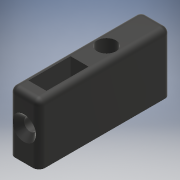
# Autodesk Inventor part: hotend__belt_holder
Saved by Autodesk Inventor 2018 (Build 220112000, 112)
## iProperties
Created: 2018-07-17
Part Number: hotend__belt_holder
Material: ABS Plastic
Document SubType Name: Modeling
Designer: Z. Deniz
Density: 1.06 g/cm^3
Appearance: Smooth - White
Author: Z. Deniz
Autodesk Inventor part; units mm, degrees
ref_plane "YZ Plane" through (0, 0, 0) normal (1, 0, 0) x (0, 1, 0)
ref_plane "XZ Plane" through (0, 0, 0) normal (0, 1, 0) x (-1, 0, 0)
ref_plane "XY Plane" through (0, 0, 0) normal (0, 0, 1) x (1, 0, 0)
sketch "Sketch1" plane through (0, 0, 0) normal (0, 0, 1) x (1, 0, 0)
  line L0 (0, 0) -> (5, 0)
  line L1 (5, 0) -> (5, 22)
  line L2 (5, 22) -> (0, 22)
  line L3 (0, 22) -> (0, 0)
  line L4 (2.5, 0) -> (2.5, 22) construction
  circle A0 centre (2.5, 13.75) radius 1.575
  line L5 (4, 2.25) -> (1, 2.25)
  line L6 (1, 2.25) -> (1, 9.25)
  line L7 (1, 9.25) -> (4, 9.25)
  line L8 (4, 9.25) -> (4, 2.25)
  dimension "d0" = 5
  dimension "d1" = 22
  dimension "d2" = 3.15
  dimension "d3" = 13.75
  dimension "d7" = 7
  dimension "d8" = 2.25
  dimension "d9" = 1
  dimension "d10" = 1
  constraints: 18 end point, 4 parallel, 2 horizontal, 2 midpoint, 2 perpendicular, 1 centre point, 1 point on line
  measures "d0" distance of L2.end L1.end
  measures "d1" distance of L1.end L0.end
  measures "d2" diameter of A0
  measures "d3" distance from line of L0 A0.centre
  measures "d7" distance of L5.end L6.end
  measures "d8" distance between parallel lines of L0 L5
  measures "d9" distance between parallel lines of L1 L8
  measures "d10" distance between parallel lines of L3 L6
extrude "Extrusion1" add sketch "Sketch1" along normal blind 10
fillet "Fillet1" radius 1 8 edges at (2.5, 22, 10) (5, 11, 10) (2.5, 0, 10) (5, 22, 5) (0, 22, 5) (5, 0, 5) (0, 0, 5) (0, 11, 10)
sketch "Sketch2" plane through (0, 0, 0) normal (0, 0, -1) x (-1, 0, 0)
  line L0 (-1, 0) -> (-4, 0) projected
  line L1 (0, 21) -> (0, 1) projected
  line L2 (-4, 22) -> (-1, 22) projected
  line L3 (-5, 1) -> (-5, 21) projected
  line L4 (-1, 9.25) -> (-1, 2.25) projected
  line L5 (-1, 2.25) -> (-4, 2.25) projected
  line L6 (-4, 2.25) -> (-4, 9.25) projected
  line L7 (-4, 9.25) -> (-1, 9.25) projected
  circle A0 centre (-2.5, 13.75) radius 1.575 projected
  arc A1 (-5, 1) -> (-4, 0) centre (-4, 1) ccw projected
  arc A2 (-1, 0) -> (0, 1) centre (-1, 1) ccw projected
  arc A3 (0, 21) -> (-1, 22) centre (-1, 21) ccw projected
  arc A4 (-4, 22) -> (-5, 21) centre (-4, 21) ccw projected
  point P0 (0, 0)
extrude "Extrusion2" add sketch "Sketch2" against normal blind 2.5 contours L4 L5 L6 L7
sketch "Sketch4" plane through (0, 0, 0) normal (0, -1, 0) x (1, 0, 0)
  line L0 (1, 0) -> (4, 0) projected
  line L1 (1, 10) -> (4, 10) construction
  line L2 (2.5, 10) -> (2.5, 0) construction
  line L3 (4.075, 0) -> (0.925, 0) construction
  circle A0 centre (2.5, 5) radius 1
  line L4 (4, 9) -> (4, 0) projected
  line L5 (1, 9) -> (4, 9) projected
  line L6 (1, 0) -> (1, 9) projected
  point P0 (0, 0)
  dimension "d13" = 2
  dimension "d14" = 5
  constraints: 3 midpoint, 2 end point, 1 centre point
  measures "d13" diameter of A0
  measures "d14" distance of L2.end A0.centre
extrude "Extrusion3" cut sketch "Sketch4" against normal blind 10.5 contours A0
chamfer "Chamfer1" distance 1 angle 45 1 edges at (1.5, 0, 5)
equation "\"d10\" = d9"
body "Solid1"
